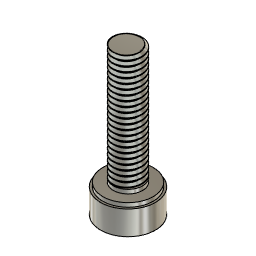
M3 x 12 v2 (Autodesk Fusion 360 design; units mm, degrees)
Autodesk Fusion 360 part; units mm, degrees
sketch "Sketch1" plane through (0, 0, 0) normal (0, 0, 1) x (1, 0, 0)
  circle A0 centre (0, 0) radius 2.74
  dimension "d1" = 5.48
  constraint coincident A0.centre origin
  measures "d1" diameter of A0
extrude "Extrude1" add sketch "Sketch1" along normal blind 2.4
sketch "Sketch2" plane through (0, 0, 2.4) normal (0, 0, 1) x (-1, 0, 0)
  circle A0 centre (0, 0) radius 2.74
  circle A1 centre (0, 0) radius 2.525
  dimension "d4" = 5.05
  constraint concentric A0 A1
  measures "d4" diameter of A1
extrude "Extrude2" add sketch "Sketch2" along normal blind 0.4 contours A1
sketch "Sketch3" plane through (0, 0, 2.8) normal (0, 0, 1) x (-1, 0, 0)
  circle A0 centre (0, 0) radius 2.525
  circle A1 centre (0, 0) radius 1.425
  dimension "d7" = 2.85
  constraint coincident A0.centre A1.centre
  measures "d7" diameter of A1
extrude "Extrude3" add sketch "Sketch3" along normal blind 12 contours A1
thread "Thread1" "ISO Metric profile 3.0 M3x0.5 6g" major diameter 2.927 minor diameter 2.3555 pitch 0.5 angle 60 modelled right hand crest width 0.0713 on face at (-1.4232, 0.071, 10.8) from (0, 0, 3.2) to (0, 0, 14.8) crest through (-1.4635, 0, 2.675)
sketch "Sketch4" plane through (0, 0, 0) normal (0, 0, -1) x (1, 0, 0)
  circle A0 centre (0, 0) radius 2.74
  line L0 (-1.5, -0.866) -> (0, -1.7321)
  line L1 (0, -1.7321) -> (1.5, -0.866)
  line L2 (1.5, -0.866) -> (1.5, 0.866)
  line L3 (1.5, 0.866) -> (0, 1.7321)
  line L4 (0, 1.7321) -> (-1.5, 0.866)
  line L5 (-1.5, 0.866) -> (-1.5, -0.866)
  dimension "d10" = 1.5
  constraint coincident A0.centre origin
  measures "d10" distance of A0.centre L5
extrude "Extrude4" cut sketch "Sketch4" against normal blind 0.8 contours L0 L1 L2 L3 L4 L5
extrude "Extrude5" cut 1 faces at (-0.5, 0.2887, 0.8) along direction (0, 0, 1) blind 0.4 draft -80
